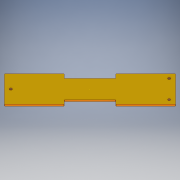
# Autodesk Inventor part: PCB-blank-20x20
Saved by Autodesk Inventor 2017 SP1 (Build 210196100, 196)
## iProperties
Created: 2017-02-03
Part Number: PCB-blank-20x20
Material: Generic
Document SubType Name: Modeling
Designer: Alex
Density: 1 g/cm^3
Appearance: Orange
Author: Alex
Autodesk Inventor part; units mm, degrees
ref_plane "YZ Plane" through (0, 0, 0) normal (1, 0, 0) x (0, 1, 0)
ref_plane "XZ Plane" through (0, 0, 0) normal (0, 1, 0) x (-1, 0, 0)
ref_plane "XY Plane" through (0, 0, 0) normal (0, 0, 1) x (1, 0, 0)
sketch "Sketch1" plane through (0, 0, 0) normal (0, 1, 0) x (-1, 0, 0)
  line L0 (10, 40) -> (-10, 40)
  line L1 (-10, -40) -> (10, -40)
  line L2 (-7, 12) -> (-7, -12)
  line L3 (7, -12) -> (7, 12)
  line L4 (7, 12) -> (10, 12)
  line L5 (7, -12) -> (10, -12)
  line L6 (-7, 12) -> (-10, 12)
  line L7 (-7, -12) -> (-10, -12)
  line L8 (-10, 40) -> (-10, 12)
  line L9 (-10, -12) -> (-10, -40)
  line L10 (10, -40) -> (10, -12)
  line L11 (10, 12) -> (10, 40)
  point P0 (0, 0)
  dimension "d0" = 20
  dimension "d1" = 80
  dimension "fullHeight" = 20
  dimension "endWidth" = 28
  dimension "d6" = 28
  dimension "midWidth" = 24
  dimension "midHeight" = 14
  constraints: 24 end point, 6 parallel, 6 perpendicular, 2 point on line, 1 horizontal
  measures "d0" distance of L1.end L1.start
  measures "d1" distance of L1.start L0.end
  measures "fullHeight" distance of L0.start L0.end
  measures "endWidth" distance of L4.end L0.start
  measures "d6" distance of L1.end L5.end
  measures "midWidth" distance of L3.start L3.end
  measures "midHeight" distance between parallel lines of L2 L3
extrude "Extrusion1" add sketch "Sketch1" along normal blind 1
sketch "Sketch2" plane through (0, 1, 0) normal (0, 1, 0) x (1, 0, 0)
  line L0 (-10, -12) -> (-10, -40) projected
  line L1 (-10, -40) -> (-10, -12) projected
  line L2 (-10, -12) -> (-7, -12) projected
  line L3 (-7, -12) -> (-7, 12) projected
  line L4 (-7, 12) -> (-10, 12) projected
  line L5 (-10, 12) -> (-10, 40) projected
  line L6 (-10, 40) -> (10, 40) projected
  line L7 (10, 40) -> (10, 12) projected
  line L8 (10, 12) -> (7, 12) projected
  line L9 (7, 12) -> (7, -12) projected
  line L10 (7, -12) -> (10, -12) projected
  line L11 (10, -12) -> (10, -40) projected
  line L12 (10, -40) -> (-10, -40) projected
  point P0 (0, 0)
extrude "Extrusion2" add sketch "Sketch2" along normal blind 0.2
sketch "Sketch6" plane through (0, 1.2, 0) normal (0, 1, 0) x (1, 0, 0)
  line L0 (-7, -37) -> (7, -37) construction
  line L1 (7, -37) -> (7, -15) construction
  line L2 (7, -15) -> (-7, -15) construction
  line L3 (-7, -15) -> (-7, -37) construction
  line L4 (-10, -12) -> (-10, -40) projected
  line L5 (-10, -40) -> (10, -40) projected
  line L6 (10, -40) -> (10, -12) projected
  line L7 (-7, 12) -> (-7, -12) projected
  line L8 (-7, 0) -> (7, 0)
  line L9 (7, -12) -> (7, 12) projected
  line L10 (-7, -12) -> (-10, -12) projected
  line L11 (0, -37) -> (0, -15) construction
  line L12 (-7, 37) -> (7, 37) construction
  line L13 (7, 37) -> (7, 15) construction
  line L14 (7, 15) -> (-7, 15) construction
  line L15 (-7, 15) -> (-7, 37) construction
  line L16 (0, 37) -> (0, 15) construction
  point P0 (0, 0)
  dimension "d18" = 3
  dimension "d19" = 3
  dimension "d27" = 3
  dimension "d28" = 3
  constraints: 22 end point, 6 symmetric about line, 4 midpoint, 2 parallel, 1 horizontal, 1 perpendicular
  measures "d18" distance between parallel lines of L5 L0
  measures "d19" distance between parallel lines of L4 L3
  measures "d27" distance between parallel lines of L6 L1
  measures "d28" distance between parallel lines of L10 L2
hole "Hole2" at (-7, 1.2, -37) at (7, 1.2, -37) at (0, 1.2, 37) direction (0, -1, 0) diameter 1.567 end through all thread size "M2x0.4" class "6H" standard "ISO Metric profile"
fillet "Fillet1" radius 0.2 12 edges at (-10, 0.6, 40) (10, 0.6, 40) (10, 0.6, -40) (-10, 0.6, -40) (10, 0.6, 12) (10, 0.6, -12) (-10, 0.6, -12) (-10, 0.6, 12) (-7, 0.6, 12) (-7, 0.6, -12) (7, 0.6, 12) (7, 0.6, -12)
equation "\"d0\" = fullHeight"
equation "\"d6\" = endWidth"
body "Solid1"
